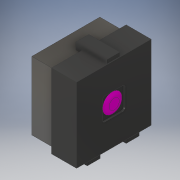
# Autodesk Inventor part: Thermal module
Saved by Autodesk Inventor 2018 (Build 220112000, 112)
## iProperties
Created: 2018-05-02
Part Number: Thermal module
Material: Generic
Document SubType Name: Modeling
Designer: Ajith Thomas
Density: 1 g/cm^3
Appearance: Default
Author: Ajith Thomas
Autodesk Inventor part; units mm, degrees
ref_plane "YZ Plane" through (0, 0, 0) normal (1, 0, 0) x (0, 1, 0)
ref_plane "XZ Plane" through (0, 0, 0) normal (0, 1, 0) x (-1, 0, 0)
ref_plane "XY Plane" through (0, 0, 0) normal (0, 0, 1) x (1, 0, 0)
sketch "Sketch1" plane through (0, 0, 0) normal (1, 0, 0) x (0, 1, 0)
  line L0 (5.75, 5.75) -> (-5.75, 5.75)
  line L1 (-5.75, 5.75) -> (-5.75, -5.75)
  line L2 (-5.75, -5.75) -> (5.75, -5.75)
  line L3 (5.75, -5.75) -> (5.75, 5.75)
  line L4 (5.75, 5.75) -> (-5.75, -5.75) construction
  line L5 (-5.75, 5.75) -> (5.75, -5.75) construction
  point P0 (0, 0)
  dimension "d0" = 11.5
  dimension "d1" = 11.5
  constraints: 12 end point, 2 midpoint, 2 parallel, 1 horizontal, 1 perpendicular
  measures "d0" distance of L2.end L1.end
  measures "d1" distance of L1.end L0.end
extrude "Extrusion1" add sketch "Sketch1" against normal blind 3.85
sketch "Sketch2" plane through (-3.85, 0, 0) normal (-1, 0, 0) x (0, 0, 1)
  line L0 (-5.25, 5.25) -> (5.25, 5.25)
  line L1 (5.25, 5.25) -> (5.25, -5.25)
  line L2 (5.25, -5.25) -> (-5.25, -5.25)
  line L3 (-5.25, -5.25) -> (-5.25, 5.25)
  line L4 (-5.25, 5.25) -> (5.25, -5.25) construction
  line L5 (5.25, 5.25) -> (-5.25, -5.25) construction
  point P0 (0, 0)
  dimension "d4" = 10.5
  dimension "d5" = 10.5
  constraints: 12 end point, 2 midpoint, 2 parallel, 1 horizontal, 1 perpendicular
  measures "d4" distance of L1.end L2.end
  measures "d5" distance of L0.end L1.end
extrude "Extrusion2" add sketch "Sketch2" along normal blind 3.56 separate body
sketch "Sketch3" plane through (-3.85, 0, 0) normal (-1, 0, 0) x (0, 0, 1)
  line L0 (5.75, 5.75) -> (-5.75, 5.75) projected
  line L1 (0, 5.75) -> (0, 5.25) construction
  line L2 (5.25, 5.25) -> (-5.25, 5.25) construction
  line L3 (0, 6.35) -> (-1, 6.35)
  line L4 (-1, 6.35) -> (-1, 5.25)
  line L5 (0, 6.35) -> (1, 6.35)
  line L6 (1, 6.35) -> (1, 5.25)
  line L7 (-1, 5.25) -> (1, 5.25) construction
  line L8 (-5.25, -5.25) -> (5.25, -5.25) projected
  line L9 (-4, -5.25) -> (-2, -5.25)
  line L10 (-2, -5.25) -> (-2, -6.35)
  line L11 (-2, -6.35) -> (-4, -6.35)
  line L12 (-4, -6.35) -> (-4, -5.25)
  line L13 (-5.25, 5.25) -> (-5.25, -5.25) projected
  line L14 (4, -5.25) -> (2, -5.25)
  line L15 (2, -5.25) -> (2, -6.35)
  line L16 (2, -6.35) -> (4, -6.35)
  line L17 (4, -6.35) -> (4, -5.25)
  line L18 (-1, 6.35) -> (1, 6.35)
  line L19 (1, 6.35) -> (1, 5.25)
  line L20 (1, 5.25) -> (-1, 5.25)
  line L21 (-1, 5.25) -> (-1, 6.35)
  point P0 (0, 0)
  dimension "d8" = 1
  dimension "d9" = 1.1
  dimension "d10" = 2
  dimension "d11" = 1.1
  dimension "d12" = 1.25
  dimension "d13" = 12.7
  constraints: 36 end point, 6 symmetric about line, 4 horizontal, 4 parallel, 3 perpendicular, 3 point on line, 2 midpoint
  measures "d8" distance of L3.start L3.end
  measures "d9" distance between parallel lines of L3 L2
  measures "d10" distance of L10.end L11.end
  measures "d11" distance of L9.end L10.end
  measures "d12" distance between parallel lines of L13 L12
  measures "d13" distance between parallel lines of L16 L5
extrude "Extrusion3" add sketch "Sketch3" along normal blind 1 and the other way blind 3.75 bodies 1
sketch "Sketch4" plane through (0, 0, 0) normal (1, 0, 0) x (0, 0, -1)
  line L0 (-1.75, 1.75) -> (1.75, 1.75)
  line L1 (1.75, 1.75) -> (1.75, -1.75)
  line L2 (1.75, -1.75) -> (-1.75, -1.75)
  line L3 (-1.75, -1.75) -> (-1.75, 1.75)
  line L4 (-1.75, 1.75) -> (1.75, -1.75) construction
  line L5 (1.75, 1.75) -> (-1.75, -1.75) construction
  point P0 (0, 0)
  dimension "d18" = 3.5
  dimension "d19" = 3.5
  constraints: 12 end point, 2 midpoint, 2 parallel, 1 horizontal, 1 perpendicular
  measures "d18" distance of L1.end L2.end
  measures "d19" distance of L0.end L1.end
extrude "Extrusion4" cut sketch "Sketch4" against normal blind 0.25 bodies 1
fillet "Fillet1" radius 0.4 4 edges at (-0.125, 1.75, 1.75) (-0.125, 1.75, -1.75) (-0.125, -1.75, 1.75) (-0.125, -1.75, -1.75)
sketch "Sketch5" plane through (-0.25, 0, 0) normal (1, 0, 0) x (0, 0, -1)
  circle A0 centre (0, 0) radius 1.5
  dimension "d23" = 3
  constraints: 1 centre point, 1 coincident
  measures "d23" diameter of A0
extrude "Extrusion5" add sketch "Sketch5" along normal blind 0.3 bodies 1
fillet "Fillet2" radius 1 1 edges at (0.05, 0, 1.5)
body "Solid1"
body "Solid2"
